Autodesk Fusion 360 part; units mm, degrees
(part 6 of 7)
  arc A999 (-78.9866, -79.4177) -> (-78.4866, -79.9177) centre (-78.4866, -79.4177) ccw
  line L1039 (33.4322, -41.8177) -> (46.4322, -41.8177)
  arc A1000 (208.3572, -60.8677) -> (208.8572, -60.3677) centre (208.3572, -60.3677) ccw
  line L1040 (-78.4866, -65.9177) -> (-65.4866, -65.9177)
  arc A1001 (-50.6991, -85.4677) -> (-51.1991, -84.9677) centre (-51.1991, -85.4677) ccw
  arc A1002 (27.3822, -41.8177) -> (27.8822, -41.3177) centre (27.3822, -41.3177) ccw
  arc A1003 (113.6072, -9.2677) -> (113.1072, -8.7677) centre (113.1072, -9.2677) ccw
  arc A1004 (-48.0303, -79.4177) -> (-47.5303, -79.9177) centre (-47.5303, -79.4177) ccw
  line L1041 (46.9322, -28.3177) -> (46.9322, -41.3177)
  arc A1005 (-20.2428, -3.7177) -> (-19.7428, -3.2177) centre (-20.2428, -3.2177) ccw
  line L1042 (4.0697, -66.4177) -> (4.0697, -79.4177)
  arc A1006 (75.7947, -60.3677) -> (76.2947, -60.8677) centre (76.2947, -60.3677) ccw
  arc A1007 (4.0697, -66.4177) -> (3.5697, -65.9177) centre (3.5697, -66.4177) ccw
  arc A1008 (194.8572, -98.4677) -> (195.3572, -98.9677) centre (195.3572, -98.4677) ccw
  line L1043 (80.5572, 9.7823) -> (80.5572, -3.2177)
  line L1044 (4.3572, 9.7823) -> (4.3572, -3.2177)
  line L1045 (27.8822, -28.3177) -> (27.8822, -41.3177)
  line L1046 (-63.0486, -66.9177) -> (-57.0486, -66.9177)
  arc A1009 (61.5072, -3.2177) -> (62.0072, -3.7177) centre (62.0072, -3.2177) ccw
  arc A1010 (-51.1991, -98.9677) -> (-50.6991, -98.4677) centre (-51.1991, -98.4677) ccw
  line L1047 (-8.9491, -86.4677) -> (-8.9491, -100.4677)
  line L1048 (175.8072, -66.4177) -> (175.8072, -79.4177)
  arc A1011 (84.5509, -85.9677) -> (84.0509, -86.4677) centre (84.5509, -86.4677) ccw
  arc A1012 (94.5572, -9.2677) -> (94.0572, -8.7677) centre (94.0572, -9.2677) ccw
  line L1049 (166.7822, -22.7677) -> (179.7822, -22.7677)
  line L1050 (176.3072, -98.9677) -> (189.3072, -98.9677)
  line L1051 (66.7697, -79.9177) -> (79.7697, -79.9177)
  line L1052 (195.3572, -60.8677) -> (208.3572, -60.8677)
  arc A1013 (-14.1928, 10.2823) -> (-14.6928, 9.7823) centre (-14.1928, 9.7823) ccw
  arc A1014 (100.1072, 10.2823) -> (99.6072, 9.7823) centre (100.1072, 9.7823) ccw
  arc A1015 (81.0572, 10.2823) -> (80.5572, 9.7823) centre (81.0572, 9.7823) ccw
  line L1053 (-0.6928, 9.7823) -> (-0.6928, -3.2177)
  line L1054 (137.7072, -9.2677) -> (137.7072, -22.2677)
  line L1055 (157.2572, -98.9677) -> (170.2572, -98.9677)
  line L1056 (179.8389, -62.8677) -> (185.8389, -62.8677)
  arc A1016 (62.0072, 10.2823) -> (61.5072, 9.7823) centre (62.0072, 9.7823) ccw
  arc A1017 (-78.4866, -65.9177) -> (-78.9866, -66.4177) centre (-78.4866, -66.4177) ccw
  line L1057 (33.4322, -27.8177) -> (46.4322, -27.8177)
  arc A1018 (-19.4553, -60.3677) -> (-18.9553, -60.8677) centre (-18.9553, -60.3677) ccw
  arc A1019 (9.6197, -65.9177) -> (9.1197, -66.4177) centre (9.6197, -66.4177) ccw
  line L1058 (84.5509, -100.9677) -> (90.5509, -100.9677)
  line L1059 (-83.2491, -60.8677) -> (-70.2491, -60.8677)
  arc A1020 (119.1572, 10.2823) -> (118.6572, 9.7823) centre (119.1572, 9.7823) ccw
  arc A1021 (-47.5303, -65.9177) -> (-48.0303, -66.4177) centre (-47.5303, -66.4177) ccw
  arc A1022 (23.4072, -22.2677) -> (23.9072, -22.7677) centre (23.9072, -22.2677) ccw
  arc A1023 (127.3947, -60.8677) -> (127.8947, -60.3677) centre (127.3947, -60.3677) ccw
  line L1060 (118.6572, -9.2677) -> (118.6572, -22.2677)
  line L1061 (62.0072, 10.2823) -> (75.0072, 10.2823)
  line L1062 (175.8072, -85.4677) -> (175.8072, -98.4677)
  line L1063 (-14.6928, 9.7823) -> (-14.6928, -3.2177)
  arc A1024 (113.8947, -60.3677) -> (114.3947, -60.8677) centre (114.3947, -60.3677) ccw
  arc A1025 (32.6447, -47.3677) -> (32.1447, -46.8677) centre (32.1447, -47.3677) ccw
  arc A1026 (185.8389, -62.8677) -> (186.3389, -62.3677) centre (185.8389, -62.3677) ccw
  line L1064 (90.0822, -28.3177) -> (90.0822, -41.3177)
  line L1065 (99.6072, -85.4677) -> (99.6072, -98.4677)
  line L1066 (195.3572, -98.9677) -> (208.3572, -98.9677)
  line L1067 (-52.2928, -8.7677) -> (-39.2928, -8.7677)
  arc A1027 (80.5572, -22.2677) -> (81.0572, -22.7677) centre (81.0572, -22.2677) ccw
  line L1068 (-14.1928, 10.2823) -> (-1.1928, 10.2823)
  arc A1028 (113.6072, 9.7823) -> (113.1072, 10.2823) centre (113.1072, 9.7823) ccw
  arc A1029 (38.1947, -46.8677) -> (37.6947, -47.3677) centre (38.1947, -47.3677) ccw
  arc A1030 (-40.3866, -84.9677) -> (-40.8866, -85.4677) centre (-40.3866, -85.4677) ccw
  line L1069 (85.3197, -66.4177) -> (85.3197, -79.4177)
  arc A1031 (132.1572, -98.9677) -> (132.6572, -98.4677) centre (132.1572, -98.4677) ccw
  arc A1032 (46.4322, -41.8177) -> (46.9322, -41.3177) centre (46.4322, -41.3177) ccw
  line L1070 (150.1134, -65.9177) -> (163.1134, -65.9177)
  line L1071 (176.3072, -79.9177) -> (189.3072, -79.9177)
  line L1072 (113.6072, -9.2677) -> (113.6072, -22.2677)
  arc A1033 (-57.5553, -60.3677) -> (-57.0553, -60.8677) centre (-57.0553, -60.3677) ccw
  arc A1034 (75.0072, -22.7677) -> (75.5072, -22.2677) centre (75.0072, -22.2677) ccw
  arc A1035 (52.4822, -27.8177) -> (51.9822, -28.3177) centre (52.4822, -28.3177) ccw
  arc A1036 (179.3389, -62.3677) -> (179.8389, -62.8677) centre (179.8389, -62.3677) ccw
  arc A1037 (113.1072, -3.7177) -> (113.6072, -3.2177) centre (113.1072, -3.2177) ccw
  arc A1038 (-38.5053, -60.3677) -> (-38.0053, -60.8677) centre (-38.0053, -60.3677) ccw
  arc A1039 (157.2572, -84.9677) -> (156.7572, -85.4677) centre (157.2572, -85.4677) ccw
  arc A1040 (94.5572, 9.7823) -> (94.0572, 10.2823) centre (94.0572, 9.7823) ccw
  arc A1041 (46.9322, -28.3177) -> (46.4322, -27.8177) centre (46.4322, -28.3177) ccw
  arc A1042 (-52.2928, 10.2823) -> (-52.7928, 9.7823) centre (-52.2928, 9.7823) ccw
  arc A1043 (-70.2491, -60.8677) -> (-69.7491, -60.3677) centre (-70.2491, -60.3677) ccw
  arc A1044 (-14.1928, -8.7677) -> (-14.6928, -9.2677) centre (-14.1928, -9.2677) ccw
  arc A1045 (189.8072, -85.4677) -> (189.3072, -84.9677) centre (189.3072, -85.4677) ccw
  arc A1046 (-34.5303, -79.9177) -> (-34.0303, -79.4177) centre (-34.5303, -79.4177) ccw
  arc A1047 (75.5072, -9.2677) -> (75.0072, -8.7677) centre (75.0072, -9.2677) ccw
  line L1073 (113.6072, 9.7823) -> (113.6072, -3.2177)
  arc A1048 (-0.6928, 9.7823) -> (-1.1928, 10.2823) centre (-1.1928, 9.7823) ccw
  arc A1049 (208.8572, -85.4677) -> (208.3572, -84.9677) centre (208.3572, -85.4677) ccw
  arc A1050 (136.9197, -79.9177) -> (137.4197, -79.4177) centre (136.9197, -79.4177) ccw
  arc A1051 (65.9822, -28.3177) -> (65.4822, -27.8177) centre (65.4822, -28.3177) ccw
  arc A1052 (75.0072, -3.7177) -> (75.5072, -3.2177) centre (75.0072, -3.2177) ccw
  arc A1053 (-15.9491, -100.4677) -> (-15.4491, -100.9677) centre (-15.4491, -100.4677) ccw
  line L1074 (114.3947, -60.8677) -> (127.3947, -60.8677)
  arc A1054 (195.3572, -84.9677) -> (194.8572, -85.4677) centre (195.3572, -85.4677) ccw
  arc A1055 (123.4197, -79.4177) -> (123.9197, -79.9177) centre (123.9197, -79.4177) ccw
  arc A1056 (-9.4303, -65.9177) -> (-9.9303, -66.4177) centre (-9.4303, -66.4177) ccw
  line L1075 (94.5572, -9.2677) -> (94.5572, -22.2677)
  line L1076 (4.3572, -9.2677) -> (4.3572, -22.2677)
  line L1077 (-74.5116, -85.4677) -> (-74.5116, -98.4677)
  arc A1057 (30.5509, -98.4677) -> (31.0509, -98.9677) centre (31.0509, -98.4677) ccw
  arc A1058 (42.4572, -22.2677) -> (42.9572, -22.7677) centre (42.9572, -22.2677) ccw
  arc A1059 (-15.4491, -85.9677) -> (-15.9491, -86.4677) centre (-15.4491, -86.4677) ccw
  line L1078 (-61.8178, -41.8177) -> (-48.8178, -41.8177)
  line L1079 (158.3442, -9.7677) -> (164.3442, -9.7677)
  line L1080 (-63.5486, -67.4177) -> (-63.5486, -81.4177)
  line L1081 (194.8572, -85.4677) -> (194.8572, -98.4677)
  line L1082 (42.1697, -66.4177) -> (42.1697, -79.4177)
  line L1083 (99.6072, 9.7823) -> (99.6072, -3.2177)
  arc A1060 (100.1072, -8.7677) -> (99.6072, -9.2677) centre (100.1072, -9.2677) ccw
  arc A1061 (-57.8428, -9.2677) -> (-58.3428, -8.7677) centre (-58.3428, -9.2677) ccw
  arc A1062 (-34.0303, -66.4177) -> (-34.5303, -65.9177) centre (-34.5303, -66.4177) ccw
  arc A1063 (-88.5116, -98.4677) -> (-88.0116, -98.9677) centre (-88.0116, -98.4677) ccw
  arc A1064 (123.9197, -65.9177) -> (123.4197, -66.4177) centre (123.9197, -66.4177) ccw
  line L1084 (75.5072, -9.2677) -> (75.5072, -22.2677)
  line L1085 (38.1947, -46.8677) -> (51.1947, -46.8677)
  arc A1065 (176.3072, -65.9177) -> (175.8072, -66.4177) centre (176.3072, -66.4177) ccw
  line L1086 (-88.0116, -84.9677) -> (-75.0116, -84.9677)
  line L1087 (-40.8866, -85.4677) -> (-40.8866, -98.4677)
  line L1088 (118.3697, -66.4177) -> (118.3697, -79.4177)
  arc A1066 (151.2072, -3.7177) -> (151.7072, -3.2177) centre (151.2072, -3.2177) ccw
  arc A1067 (22.6197, -79.9177) -> (23.1197, -79.4177) centre (22.6197, -79.4177) ccw
  arc A1068 (-80.4246, -67.4177) -> (-80.9246, -66.9177) centre (-80.9246, -67.4177) ccw
  line L1089 (18.3572, -9.2677) -> (18.3572, -22.2677)
  line L1090 (-26.8866, -85.4677) -> (-26.8866, -98.4677)
  arc A1069 (155.4629, -62.3677) -> (155.9629, -62.8677) centre (155.9629, -62.3677) ccw
  arc A1070 (119.1572, -8.7677) -> (118.6572, -9.2677) centre (119.1572, -9.2677) ccw
  arc A1071 (-39.2928, -3.7177) -> (-38.7928, -3.2177) centre (-39.2928, -3.2177) ccw
  line L1091 (31.0509, -98.9677) -> (44.0509, -98.9677)
  line L1092 (-64.9866, -66.4177) -> (-64.9866, -79.4177)
  line L1093 (-87.4246, -67.4177) -> (-87.4246, -81.4177)
  arc A1072 (17.8572, -22.7677) -> (18.3572, -22.2677) centre (17.8572, -22.2677) ccw
  arc A1073 (-83.7491, -60.3677) -> (-83.2491, -60.8677) centre (-83.2491, -60.3677) ccw
  arc A1074 (108.3447, -60.8677) -> (108.8447, -60.3677) centre (108.3447, -60.3677) ccw
  line L1094 (176.3072, -65.9177) -> (189.3072, -65.9177)
  line L1095 (151.7072, 9.7823) -> (151.7072, -3.2177)
  line L1096 (-15.9491, -86.4677) -> (-15.9491, -100.4677)
  arc A1075 (-52.2928, -8.7677) -> (-52.7928, -9.2677) centre (-52.2928, -9.2677) ccw
  line L1097 (-15.4491, -100.9677) -> (-9.4491, -100.9677)
  line L1098 (44.5509, -85.4677) -> (44.5509, -98.4677)
  arc A1076 (57.2447, -46.8677) -> (56.7447, -47.3677) centre (57.2447, -47.3677) ccw
  arc A1077 (85.3197, -79.4177) -> (85.8197, -79.9177) centre (85.8197, -79.4177) ccw
  line L1099 (-48.0303, -66.4177) -> (-48.0303, -79.4177)
  line L1100 (80.5572, -9.2677) -> (80.5572, -22.2677)
  arc A1078 (-15.4803, -79.9177) -> (-14.9803, -79.4177) centre (-15.4803, -79.4177) ccw
  line L1101 (56.4572, -9.2677) -> (56.4572, -22.2677)
  line L1102 (138.2072, 10.2823) -> (151.2072, 10.2823)
  arc A1079 (-74.5116, -85.4677) -> (-75.0116, -84.9677) centre (-75.0116, -85.4677) ccw
  line L1103 (156.7572, 9.7823) -> (156.7572, -3.2177)
  line L1104 (47.2197, -66.4177) -> (47.2197, -79.4177)
  arc A1080 (9.1197, -79.4177) -> (9.6197, -79.9177) centre (9.6197, -79.4177) ccw
  arc A1081 (44.0509, -98.9677) -> (44.5509, -98.4677) centre (44.0509, -98.4677) ccw
  line L1105 (-50.6991, -85.4677) -> (-50.6991, -98.4677)
  arc A1082 (118.6572, -3.2177) -> (119.1572, -3.7177) centre (119.1572, -3.2177) ccw
  line L1106 (100.1072, -8.7677) -> (113.1072, -8.7677)
  line L1107 (104.3697, -66.4177) -> (104.3697, -79.4177)
  arc A1083 (4.8572, -8.7677) -> (4.3572, -9.2677) centre (4.8572, -9.2677) ccw
  line L1108 (186.3389, -48.3677) -> (186.3389, -62.3677)
  arc A1084 (99.6072, -3.2177) -> (100.1072, -3.7177) centre (100.1072, -3.2177) ccw
  arc A1085 (118.3697, -66.4177) -> (117.8697, -65.9177) centre (117.8697, -66.4177) ccw
  line L1109 (28.6697, -65.9177) -> (41.6697, -65.9177)
  arc A1086 (60.7197, -79.9177) -> (61.2197, -79.4177) centre (60.7197, -79.4177) ccw
  arc A1087 (151.7072, 9.7823) -> (151.2072, 10.2823) centre (151.2072, 9.7823) ccw
  arc A1088 (51.1947, -60.8677) -> (51.6947, -60.3677) centre (51.1947, -60.3677) ccw
  arc A1089 (117.8697, -79.9177) -> (118.3697, -79.4177) centre (117.8697, -79.4177) ccw
  arc A1090 (-40.8866, -98.4677) -> (-40.3866, -98.9677) centre (-40.3866, -98.4677) ccw
  arc A1091 (-33.2428, 10.2823) -> (-33.7428, 9.7823) centre (-33.2428, 9.7823) ccw
  arc A1092 (66.2697, -79.4177) -> (66.7697, -79.9177) centre (66.7697, -79.4177) ccw
  line L1110 (157.2572, 10.2823) -> (170.2572, 10.2823)
  arc A1093 (176.3072, -84.9677) -> (175.8072, -85.4677) centre (176.3072, -85.4677) ccw
  arc A1094 (-64.1991, -84.9677) -> (-64.6991, -85.4677) centre (-64.1991, -85.4677) ccw
  arc A1095 (-64.9866, -66.4177) -> (-65.4866, -65.9177) centre (-65.4866, -66.4177) ccw
  line L1111 (-80.4246, -67.4177) -> (-80.4246, -81.4177)
  arc A1096 (3.5697, -79.9177) -> (4.0697, -79.4177) centre (3.5697, -79.4177) ccw
  arc A1097 (-58.3428, -3.7177) -> (-57.8428, -3.2177) centre (-58.3428, -3.2177) ccw
  arc A1098 (-28.4803, -65.9177) -> (-28.9803, -66.4177) centre (-28.4803, -66.4177) ccw
  line L1112 (100.1072, -3.7177) -> (113.1072, -3.7177)
  arc A1099 (-5.9553, -60.8677) -> (-5.4553, -60.3677) centre (-5.9553, -60.3677) ccw
  arc A1100 (-88.0116, -84.9677) -> (-88.5116, -85.4677) centre (-88.0116, -85.4677) ccw
  line L1113 (37.4072, -9.2677) -> (37.4072, -22.2677)
  arc A1101 (51.6947, -47.3677) -> (51.1947, -46.8677) centre (51.1947, -47.3677) ccw
  arc A1102 (19.1447, -46.8677) -> (18.6447, -47.3677) centre (19.1447, -47.3677) ccw
  arc A1103 (51.9822, -41.3177) -> (52.4822, -41.8177) centre (52.4822, -41.3177) ccw
  line L1114 (99.3197, -66.4177) -> (99.3197, -79.4177)
  line L1115 (-19.7428, -9.2677) -> (-19.7428, -22.2677)
  line L1116 (-103.7226, 22.4007) -> (218.9474, 22.4007)
  line L1117 (218.9474, 22.4007) -> (218.9474, -108.8427)
  line L1118 (218.9474, -108.8427) -> (-103.7226, -108.8427)
  line L1119 (-103.7226, -108.8427) -> (-103.7226, 22.4007)
  circle A1104 centre (-107.7226, 51.4273) radius 1.75
  circle A1105 centre (-107.7226, -112.8427) radius 1.75
  circle A1106 centre (222.9474, 51.4273) radius 1.75
  circle A1107 centre (222.9474, -112.8427) radius 1.75
  dimension "d1" = 25.211
  dimension "d2" = 19.875
  dimension "d3" = 25.211
  dimension "d4" = 19.875
  dimension "d5" = 25.211
  dimension "d6" = 19.875
  dimension "d8" = 10
  dimension "d9" = 10
  dimension "d10" = 10
  dimension "d11" = 3.5
  dimension "d12" = 6
  dimension "d13" = 6
  dimension "d14" = 3.5
  dimension "d15" = 6
  dimension "d16" = 6
  dimension "d17" = 3.5
  dimension "d18" = 6
  dimension "d19" = 6
  dimension "d20" = 3.5
  dimension "d21" = 6
  dimension "d22" = 6
  constraint horizontal L40
  constraint vertical L60
  constraint horizontal L155
  constraint vertical L18
  constraint horizontal L412
  constraint vertical L432
  constraint horizontal L527
  constraint vertical L390
  constraint horizontal L784
  constraint vertical L804
  constraint horizontal L899
  constraint vertical L762
  constraint horizontal L1116
  constraint vertical L1117
  constraint horizontal L1118
  constraint vertical L1119
  measures "d1" distance of L18 L112
  measures "d2" distance of L100 L155
  measures "d3" distance of L390 L484
  measures "d4" distance of L472 L527
  measures "d5" distance of L762 L856
  measures "d6" distance of L844 L899
  measures "d8" distance of L762 L1119
  measures "d9" distance of L804 L1117
  measures "d10" distance of L527 L1118
  measures "d11" diameter of A1107
  measures "d12" distance of L804 A1107.centre
  measures "d13" distance of L899 A1107.centre
  measures "d14" diameter of A1106
  measures "d15" distance of L60 A1106.centre
  measures "d16" distance of L784 A1106.centre
  measures "d17" diameter of A1104
  measures "d18" distance of L412 A1104.centre
  measures "d19" distance of L762 A1104.centre
  measures "d20" diameter of A1105
  measures "d21" distance of L527 A1105.centre
  measures "d22" distance of L18 A1105.centre
extrude "Extrude1" add sketch "Sketch1" along normal blind 6 contours L18 L40 L60 L155 L390 L412 L432 L527 L762 L784 L804 L899 makes body 1
fillet "Fillet1" radius 9 4 edges at (-113.7226, -118.8427, 3) (-113.7226, 57.4273, 3) (228.9474, 57.4273, 3) (228.9474, -118.8427, 3) on bodies 1
fillet "Fillet2" radius 5 4 edges at (218.9474, 22.4007, 3) (-103.7226, 22.4007, 3) (-103.7226, -108.8427, 3) (218.9474, -108.8427, 3) on bodies 1
sketch "Sketch2" plane through (0, 0, 6) normal (0, 0, 1) x (-1, 0, 0)
  arc A0 (-219.9474, 118.8427) -> (-228.9474, 109.8427) centre (-219.9474, 109.8427) ccw
  line L0 (-228.9474, 109.8427) -> (-228.9474, -48.4273)
  arc A1 (-228.9474, -48.4273) -> (-219.9474, -57.4273) centre (-219.9474, -48.4273) ccw
  line L1 (-219.9474, -57.4273) -> (104.7226, -57.4273)
  arc A2 (104.7226, -57.4273) -> (113.7226, -48.4273) centre (104.7226, -48.4273) ccw
  line L2 (113.7226, -48.4273) -> (113.7226, 109.8427)
  arc A3 (113.7226, 109.8427) -> (104.7226, 118.8427) centre (104.7226, 109.8427) ccw
  line L3 (104.7226, 118.8427) -> (-219.9474, 118.8427)
  circle A4 centre (107.7226, 112.8427) radius 1.75
  circle A5 centre (-222.9474, 112.8427) radius 1.75
  circle A6 centre (-222.9474, -51.4273) radius 1.75
  line L4 (-213.9474, 108.8427) -> (98.7226, 108.8427)
  arc A7 (103.7226, 103.8427) -> (98.7226, 108.8427) centre (98.7226, 103.8427) ccw
  line L5 (103.7226, 103.8427) -> (103.7226, -17.4007)
  arc A8 (98.7226, -22.4007) -> (103.7226, -17.4007) centre (98.7226, -17.4007) ccw
  line L6 (98.7226, -22.4007) -> (-213.9474, -22.4007)
  arc A9 (-218.9474, -17.4007) -> (-213.9474, -22.4007) centre (-213.9474, -17.4007) ccw
  line L7 (-218.9474, -17.4007) -> (-218.9474, 103.8427)
  arc A10 (-213.9474, 108.8427) -> (-218.9474, 103.8427) centre (-213.9474, 103.8427) ccw
  circle A11 centre (107.7226, -51.4273) radius 1.75
  line L8 (110, -40) -> (110, 105)
  line L9 (108, 105) -> (108, 96)
  line L10 (108, 96) -> (106.5, 95)
  line L11 (106.5, 95) -> (106.5, 90)
  line L12 (106.5, 90) -> (108, 88.6859)
  line L13 (108, 88.6859) -> (108, 59)
  line L14 (108, 59) -> (106, 58)
  line L15 (106, 58) -> (106, 28)
  line L16 (106, 28) -> (108, 24)
  line L17 (108, 24) -> (108, -19)
  line L18 (108, -19) -> (107, -21)
  line L19 (107, -21) -> (105, -21)
  line L20 (105, -21) -> (104, -23)
  line L21 (104, -23) -> (102, -23)
  line L22 (102, -23) -> (101, -25)
  line L23 (101, -25) -> (97, -25)
  line L24 (97, -25) -> (95, -27)
  line L25 (95, -27) -> (95, -30)
  line L26 (95, -30) -> (95, -37.2329)
  line L27 (95, -37.2329) -> (94.9816, -37.2145)
  line L28 (110, -40) -> (110, -45)
  line L29 (110, -45) -> (107, -46)
  line L30 (107, -46) -> (104.7226, -46.7591)
  line L31 (104.7226, -46.7591) -> (99.718, -48.4273)
  line L32 (99.718, -48.4273) -> (99.718, -51)
  line L33 (99.718, -51) -> (55, -51)
  line L34 (55, -51) -> (53.023, -52.318)
  line L35 (53.023, -52.318) -> (24.5454, -52.318)
  line L36 (24.5454, -52.318) -> (23.6667, -51)
  line L37 (23.6667, -51) -> (-31, -51)
  line L38 (-31, -51) -> (-80, -51)
  line L39 (-80, -51) -> (-83, -54)
  line L40 (-83, -54) -> (-120, -54)
  line L41 (-120, -54) -> (-122, -51)
  line L42 (-122, -51) -> (-200, -51)
  line L43 (-200, -51) -> (-204.3677, -48.4273)
  line L44 (-204.3677, -48.4273) -> (-209, -48.4273)
  line L45 (-209, -48.4273) -> (-212.364, -46.4459)
  line L46 (-212.364, -46.4459) -> (-216, -46.4459)
  line L47 (-216, -46.4459) -> (-218.7538, -44.8239)
  line L48 (-218.7538, -44.8239) -> (-223, -44.8239)
  line L49 (-223, -44.8239) -> (-224.9863, -43.6539)
  line L50 (-224.9863, -43.6539) -> (-224.9863, -21)
  line L51 (-224.9863, -21) -> (-227, -19)
  line L52 (-227, -19) -> (-227, -10)
  line L53 (-227, -10) -> (-224.9863, -6.5812)
  line L54 (-224.9863, -6.5812) -> (-224.9863, 40)
  line L55 (-224.9863, 40) -> (-227, 43.4506)
  line L56 (-227, 43.4506) -> (-227, 75)
  line L57 (-227, 75) -> (-224.9863, 77.9634)
  line L58 (-224.9863, 77.9634) -> (-224.9863, 105)
  line L59 (-224.9863, 105) -> (-224.9863, 107.3782)
  line L60 (-224.9863, 107.3782) -> (-222, 108)
  line L61 (-222, 108) -> (-219.9474, 109.8427)
  line L62 (-219.9474, 109.8427) -> (-217.5, 112.5)
  line L63 (-217.5, 112.5) -> (-215, 115)
  line L64 (-215, 115) -> (-111.4311, 115)
  line L65 (-111.4311, 115) -> (-99, 115)
  line L66 (-99, 115) -> (-97.0321, 116.7667)
  line L67 (-97.0321, 116.7667) -> (-32.7128, 116.7667)
  line L68 (-32.7128, 116.7667) -> (-30, 115)
  line L69 (-30, 115) -> (100, 115)
  line L70 (100, 115) -> (102.1243, 112.8427)
  line L71 (102.1243, 112.8427) -> (104.0883, 112.4123)
  line L72 (104.0883, 112.4123) -> (105.5565, 110.9212)
  line L73 (105.5565, 110.9212) -> (107.1244, 109.329)
  line L74 (107.1244, 109.329) -> (110, 109.329)
  line L75 (110, 109.329) -> (110, 105)
  line L76 (108, 105) -> (108, 107)
  line L77 (108, 107) -> (105, 107)
  line L78 (105, 107) -> (103, 110)
  line L79 (103, 110) -> (101, 111)
  line L80 (101, 111) -> (98.9961, 113.0039)
  line L81 (98.9961, 113.0039) -> (78.0039, 113.0039)
  line L82 (78.0039, 113.0039) -> (76, 111)
  line L83 (76, 111) -> (58, 111)
  line L84 (58, 111) -> (56, 113)
  line L85 (56, 113) -> (12, 113)
  line L86 (12, 113) -> (10, 111)
  line L87 (10, 111) -> (0, 111)
  line L88 (0, 111) -> (-2, 113)
  line L89 (-2, 113) -> (-105, 113)
  line L90 (-105, 113) -> (-140, 113)
  line L91 (-140, 113) -> (-195, 113)
  line L92 (-195, 113) -> (-197, 111)
  line L93 (-197, 111) -> (-206, 111)
  line L94 (-206, 111) -> (-207.5, 112.5)
  line L95 (-207.5, 112.5) -> (-208, 113)
  line L96 (-208, 113) -> (-214, 113)
  line L97 (-214, 113) -> (-215, 113)
  line L98 (-215, 113) -> (-218.9474, 109.0526)
  line L99 (-218.9474, 109.0526) -> (-221.3805, 106.6195)
  line L100 (-221.3805, 106.6195) -> (-223, 106)
  line L101 (-223, 106) -> (-223, 35)
  line L102 (-223, 35) -> (-222, 34)
  line L103 (-222, 34) -> (-222, 8.6485)
  line L104 (-222, 8.6485) -> (-223, 7)
  line L105 (-223, 7) -> (-223, -36.5124)
  line L106 (-223, -36.5124) -> (-218.7538, -40.3244)
  line L107 (-218.7538, -40.3244) -> (-214.9132, -42.5866)
  line L108 (-214.9132, -42.5866) -> (-209, -42.5866)
  line L109 (-209, -42.5866) -> (-206.5079, -44.8239)
  line L110 (-206.5079, -44.8239) -> (-203, -44.8239)
  line L111 (-203, -44.8239) -> (-198, -49)
  line L112 (-198, -49) -> (-166, -49)
  line L113 (-166, -49) -> (-164.1255, -46.9119)
  line L114 (-164.1255, -46.9119) -> (-144, -46.9119)
  line L115 (-144, -46.9119) -> (-141.6741, -49)
  line L116 (-141.6741, -49) -> (-55, -49)
  line L117 (-55, -49) -> (-53.1255, -46.9119)
  line L118 (-53.1255, -46.9119) -> (-7, -46.9119)
  line L119 (-7, -46.9119) -> (-5, -49)
  line L120 (-5, -49) -> (90.0217, -49)
  line L121 (90.0217, -49) -> (95.0077, -45.5)
  line L122 (95.0077, -45.5) -> (95.0077, -45.4411)
  line L123 (95.0077, -45.4411) -> (94.9816, -37.2145)
  line L124 (79.9728, -47.0166) -> (85.4987, -44.6483)
  line L125 (85.4987, -44.6483) -> (85.4987, -43.6179)
  line L126 (85.4987, -43.6179) -> (79.9839, -45.9814)
  line L127 (79.9728, -47.0166) -> (79.9839, -45.9814) construction
  line L128 (79.9728, -47.0166) -> (74.4988, -44.5304)
  line L129 (74.4988, -44.5304) -> (74.5209, -43.5002)
  line L130 (74.5209, -43.5002) -> (79.9839, -45.9814)
  line L131 (80.0522, -44.5759) -> (74.5262, -42.2076)
  line L132 (80.0522, -44.5759) -> (85.5261, -42.0897)
  line L133 (85.504, -41.0595) -> (80.0411, -43.5407)
  line L134 (85.5261, -42.0897) -> (85.504, -41.0595)
  line L135 (74.5262, -41.1772) -> (80.0411, -43.5407)
  line L136 (74.5262, -42.2076) -> (74.5262, -41.1772)
  line L137 (79.9047, -39.8001) -> (74.4308, -37.3139)
  line L138 (85.4307, -37.4319) -> (85.4307, -36.4015)
  line L139 (79.9047, -39.8001) -> (85.4307, -37.4319)
  line L140 (85.4581, -39.7547) -> (85.436, -38.7245)
  line L141 (74.4308, -37.3139) -> (74.4529, -36.2838)
  line L142 (85.436, -38.7245) -> (79.9731, -41.2057)
  line L143 (74.4529, -36.2838) -> (79.9158, -38.765)
  line L144 (79.9842, -42.2409) -> (85.4581, -39.7547)
  line L145 (74.4582, -39.8726) -> (74.4582, -38.8422)
  line L146 (85.4307, -36.4015) -> (79.9158, -38.765)
  line L147 (79.9842, -42.2409) -> (74.4582, -39.8726)
  line L148 (79.9842, -42.2409) -> (79.9731, -41.2057) construction
  line L149 (74.4582, -38.8422) -> (79.9731, -41.2057)
  line L150 (85.4987, -47.4996) -> (85.4987, -25.2234) construction
  line L151 (79.8932, -32.8108) -> (79.9043, -31.7757) construction
  line L152 (74.3733, -31.6295) -> (79.8362, -34.1107)
  line L153 (74.3786, -35.2183) -> (74.3786, -34.1879)
  line L154 (79.8251, -35.1458) -> (85.3511, -32.7776)
  line L155 (74.3786, -34.1879) -> (79.8935, -36.5514)
  line L156 (79.8932, -32.8108) -> (74.4193, -30.3246)
  line L157 (74.3512, -32.6596) -> (74.3733, -31.6295)
  line L158 (79.9046, -37.5866) -> (85.3785, -35.1004)
  line L159 (79.8932, -32.8108) -> (85.4192, -30.4426)
  line L160 (85.3511, -31.7472) -> (79.8362, -34.1107)
  line L161 (85.3511, -32.7776) -> (85.3511, -31.7472)
  line L162 (79.9046, -37.5866) -> (79.8935, -36.5514) construction
  line L163 (85.4192, -30.4426) -> (85.4192, -29.4122)
  line L164 (74.4414, -29.2945) -> (79.9043, -31.7757)
  line L165 (85.3785, -35.1004) -> (85.3564, -34.0702)
  line L166 (74.4467, -26.9714) -> (79.9615, -29.335)
  line L167 (79.9726, -30.3701) -> (74.4467, -28.0018)
  line L168 (79.8251, -35.1458) -> (74.3512, -32.6596)
  line L169 (85.4466, -27.8839) -> (85.4245, -26.8538)
  line L170 (85.3564, -34.0702) -> (79.8935, -36.5514)
  line L171 (79.9046, -37.5866) -> (74.3786, -35.2183)
  line L172 (79.9726, -30.3701) -> (85.4466, -27.8839)
  line L173 (85.4245, -26.8538) -> (79.9615, -29.335)
  line L174 (74.4193, -30.3246) -> (74.4414, -29.2945)
  line L175 (85.4192, -29.4122) -> (79.9043, -31.7757)
  line L176 (74.4467, -28.0018) -> (74.4467, -26.9714)
  line L177 (55, -46) -> (65, -30)
  line L178 (65, -30) -> (44, -30)
  line L179 (44, -30) -> (55, -46)
  line L180 (55, -48) -> (67, -29)
  line L181 (67, -29) -> (42, -29)
  line L182 (42, -29) -> (55, -48)
  line L183 (55.638, -43.2362) -> (54.2071, -43.2362)
  line L184 (54.2071, -43.2362) -> (54.2071, -33.9141)
  line L185 (54.2071, -33.9141) -> (55.638, -33.9141)
  line L186 (55.638, -33.9141) -> (55.638, -43.2362)
  circle A12 centre (54.9514, -32.4983) radius 0.8407
  line L187 (-144.2264, -40.7236) -> (-140.2264, -36.7236)
  line L188 (-140.2264, -36.7236) -> (-179.2264, -36.7236)
  line L189 (-179.2264, -36.7236) -> (-180.0146, -38.3)
  line L190 (-180.0146, -38.3) -> (-152.9, -38.3)
  line L191 (-152.9, -38.3) -> (-151.2264, -40.7236)
  line L192 (-151.2264, -40.7236) -> (-144.2264, -40.7236)
  line L193 (-153.2344, -39.0462) -> (-189.9389, -39.1613)
  line L194 (-189.9389, -39.1613) -> (-188.2093, -42.0152)
  line L195 (-188.2093, -42.0152) -> (-151.3887, -42.0152)
  line L196 (-151.3887, -42.0152) -> (-153.2344, -39.0462)
  line L197 (-137.6491, -35) -> (-178.2775, -35)
  line L198 (-178.2775, -35) -> (-182.1257, -37.5655)
  line L199 (-182.1257, -37.5655) -> (-200, -37.5655)
  line L200 (-200, -37.5655) -> (-200, -36.377)
  line L201 (-200, -36.377) -> (-182.5655, -36.377)
  line L202 (-182.5655, -36.377) -> (-179, -34)
  line L203 (-179, -34) -> (-138.1989, -34)
  line L204 (-138.1989, -34) -> (-135.1886, -29.1904)
  line L205 (-137.6491, -35) -> (-134.2833, -29.7167)
  line L206 (-134.2833, -29.7167) -> (-135.1886, -29.1904)
  line L207 (-143.8469, -32.9977) -> (-144.4496, -32.6498)
  line L208 (-144.4496, -32.6498) -> (-142.2994, -28.9256)
  line L209 (-142.2994, -28.9256) -> (-141.6968, -29.2736)
  line L210 (-141.6968, -29.2736) -> (-143.8469, -32.9977)
  line L211 (-142.2994, -28.9256) -> (-141.6968, -29.2736)
  line L212 (-144.4496, -32.6498) -> (-142.2994, -28.9256)
  line L213 (-141.6968, -29.2736) -> (-143.8469, -32.9977)
  line L214 (-143.8469, -32.9977) -> (-144.4496, -32.6498)
  line L215 (-143.3648, -29.2464) -> (-145.5149, -32.9705)
  line L216 (-143.9674, -28.8984) -> (-143.3648, -29.2464)
  line L217 (-143.9674, -28.8984) -> (-143.3648, -29.2464)
  line L218 (-143.3648, -29.2464) -> (-145.5149, -32.9705)
  line L219 (-145.5149, -32.9705) -> (-146.1175, -32.6226)
  line L220 (-146.1175, -32.6226) -> (-143.9674, -28.8984)
  line L221 (-146.5557, -29.2101) -> (-148.7058, -32.9343)
  line L222 (-144.8877, -29.2373) -> (-147.0378, -32.9615)
  line L223 (-145.4904, -28.8894) -> (-144.8877, -29.2373)
  line L224 (-147.6405, -32.6135) -> (-145.4904, -28.8894)
  line L225 (-145.4904, -28.8894) -> (-144.8877, -29.2373)
  line L226 (-147.0378, -32.9615) -> (-147.6405, -32.6135)
  line L227 (-147.0378, -32.9615) -> (-147.6405, -32.6135)
  line L228 (-144.8877, -29.2373) -> (-147.0378, -32.9615)
  line L229 (-147.1583, -28.8622) -> (-146.5557, -29.2101)
  line L230 (-147.1583, -28.8622) -> (-146.5557, -29.2101)
  line L231 (-147.6405, -32.6135) -> (-145.4904, -28.8894)
  line L232 (-146.5557, -29.2101) -> (-148.7058, -32.9343)
  line L233 (-148.7058, -32.9343) -> (-149.3085, -32.5863)
  line L234 (-149.3085, -32.5863) -> (-147.1583, -28.8622)
  line L235 (-152.7417, -32.59) -> (-150.5916, -28.8659)
  line L236 (-150.4711, -32.9652) -> (-151.0737, -32.6172)
  line L237 (-153.7825, -28.8297) -> (-153.1799, -29.1776)
  line L238 (-151.0737, -32.6172) -> (-148.9236, -28.8931)
  line L239 (-149.9889, -29.2139) -> (-152.1391, -32.938)
  line L240 (-150.5916, -28.8659) -> (-149.9889, -29.2139)
  line L241 (-150.5916, -28.8659) -> (-149.9889, -29.2139)
  line L242 (-152.1391, -32.938) -> (-152.7417, -32.59)
  line L243 (-155.33, -32.9017) -> (-155.9326, -32.5538)
  line L244 (-153.662, -32.9289) -> (-154.2647, -32.581)
  line L245 (-153.662, -32.9289) -> (-154.2647, -32.581)
  line L246 (-155.9326, -32.5538) -> (-153.7825, -28.8297)
  line L247 (-150.4711, -32.9652) -> (-151.0737, -32.6172)
  line L248 (-149.9889, -29.2139) -> (-152.1391, -32.938)
  line L249 (-151.0737, -32.6172) -> (-148.9236, -28.8931)
  line L250 (-153.7825, -28.8297) -> (-153.1799, -29.1776)
  line L251 (-153.1799, -29.1776) -> (-155.33, -32.9017)
  line L252 (-152.1145, -28.8569) -> (-151.5119, -29.2048)
  line L253 (-154.2647, -32.581) -> (-152.1145, -28.8569)
  line L254 (-154.2647, -32.581) -> (-152.1145, -28.8569)
  line L255 (-152.1145, -28.8569) -> (-151.5119, -29.2048)
  line L256 (-151.5119, -29.2048) -> (-153.662, -32.9289)
  line L257 (-153.1799, -29.1776) -> (-155.33, -32.9017)
  line L258 (-151.5119, -29.2048) -> (-153.662, -32.9289)
  line L259 (-148.321, -29.2411) -> (-150.4711, -32.9652)
  line L260 (-148.9236, -28.8931) -> (-148.321, -29.2411)
  line L261 (-160.2369, -28.8156) -> (-159.6342, -29.1636)
  line L262 (-165.1931, -28.8103) -> (-164.5904, -29.1582)
  line L263 (-166.7405, -32.8824) -> (-167.3432, -32.5344)
  line L264 (-166.8611, -28.7831) -> (-166.2584, -29.131)
  line L265 (-166.8611, -28.7831) -> (-166.2584, -29.131)
  line L266 (-161.7843, -32.8877) -> (-162.387, -32.5397)
  line L267 (-159.6342, -29.1636) -> (-161.7843, -32.8877)
  line L268 (-166.2584, -29.131) -> (-168.4085, -32.8552)
  line L269 (-156.9254, -32.9511) -> (-157.5281, -32.6032)
  line L270 (-158.5689, -28.8428) -> (-157.9662, -29.1908)
  line L271 (-157.9662, -29.1908) -> (-160.1164, -32.9149)
  line L272 (-159.6342, -29.1636) -> (-161.7843, -32.8877)
  line L273 (-160.1164, -32.9149) -> (-160.719, -32.5669)
  line L274 (-157.9662, -29.1908) -> (-160.1164, -32.9149)
  line L275 (-163.6701, -28.8193) -> (-163.0675, -29.1673)
  line L276 (-156.4433, -29.1998) -> (-158.5934, -32.9239)
  line L277 (-163.5496, -32.9186) -> (-164.1523, -32.5707)
  line L278 (-166.7405, -32.8824) -> (-167.3432, -32.5344)
  line L279 (-167.3432, -32.5344) -> (-165.1931, -28.8103)
  line L280 (-156.9254, -32.9511) -> (-157.5281, -32.6032)
  line L281 (-166.2584, -29.131) -> (-168.4085, -32.8552)
  line L282 (-167.3432, -32.5344) -> (-165.1931, -28.8103)
  line L283 (-157.5281, -32.6032) -> (-155.378, -28.8791)
  line L284 (-164.1523, -32.5707) -> (-162.0021, -28.8465)
  line L285 (-161.3995, -29.1945) -> (-163.5496, -32.9186)
  line L286 (-165.1931, -28.8103) -> (-164.5904, -29.1582)
  line L287 (-169.0112, -32.5072) -> (-166.8611, -28.7831)
  line L288 (-165.2176, -32.8914) -> (-165.8203, -32.5435)
  line L289 (-163.5496, -32.9186) -> (-164.1523, -32.5707)
  line L290 (-164.5904, -29.1582) -> (-166.7405, -32.8824)
  line L291 (-165.8203, -32.5435) -> (-163.6701, -28.8193)
  line L292 (-163.0675, -29.1673) -> (-165.2176, -32.8914)
  line L293 (-160.719, -32.5669) -> (-158.5689, -28.8428)
  line L294 (-160.719, -32.5669) -> (-158.5689, -28.8428)
  line L295 (-160.2369, -28.8156) -> (-159.6342, -29.1636)
  line L296 (-168.4085, -32.8552) -> (-169.0112, -32.5072)
  line L297 (-157.046, -28.8519) -> (-156.4433, -29.1998)
  line L298 (-157.5281, -32.6032) -> (-155.378, -28.8791)
  line L299 (-160.1164, -32.9149) -> (-160.719, -32.5669)
  line L300 (-164.1523, -32.5707) -> (-162.0021, -28.8465)
  line L301 (-158.5934, -32.9239) -> (-159.1961, -32.576)
  line L302 (-164.5904, -29.1582) -> (-166.7405, -32.8824)
  line L303 (-157.046, -28.8519) -> (-156.4433, -29.1998)
  line L304 (-156.4433, -29.1998) -> (-158.5934, -32.9239)
  line L305 (-159.1961, -32.576) -> (-157.046, -28.8519)
  line L306 (-162.387, -32.5397) -> (-160.2369, -28.8156)
  line L307 (-163.0675, -29.1673) -> (-165.2176, -32.8914)
  line L308 (-163.6701, -28.8193) -> (-163.0675, -29.1673)
  line L309 (-158.5689, -28.8428) -> (-157.9662, -29.1908)
  line L310 (-162.0021, -28.8465) -> (-161.3995, -29.1945)
  line L311 (-154.7753, -29.227) -> (-156.9254, -32.9511)
  line L312 (-155.378, -28.8791) -> (-154.7753, -29.227)
  line L313 (-180.4144, -32.4692) -> (-178.2643, -28.7451)
  line L314 (-178.2643, -28.7451) -> (-177.6617, -29.0931)
  line L315 (-182.0824, -32.4421) -> (-179.9323, -28.7179)
  line L316 (-171.6401, -28.7777) -> (-171.0375, -29.1256)
  line L317 (-190.7402, -29.0465) -> (-192.8903, -32.7706)
  line L318 (-193.493, -32.4227) -> (-191.3428, -28.6985)
  line L319 (-172.2673, -32.5108) -> (-170.1172, -28.7867)
  line L320 (-169.5145, -29.1347) -> (-171.6647, -32.8588)
  line L321 (-169.5145, -29.1347) -> (-171.6647, -32.8588)
  line L322 (-177.2235, -32.5055) -> (-175.0734, -28.7814)
  line L323 (-176.1387, -29.1021) -> (-178.2888, -32.8263)
  line L324 (-188.5368, -32.428) -> (-186.3866, -28.7039)
  line L325 (-175.4582, -32.4746) -> (-173.3081, -28.7505)
  line L326 (-174.4707, -29.1293) -> (-176.6209, -32.8535)
  line L327 (-186.8688, -32.4552) -> (-184.7187, -28.7311)
  line L328 (-178.2643, -28.7451) -> (-177.6617, -29.0931)
  line L329 (-169.9967, -32.886) -> (-170.5993, -32.538)
  line L330 (-174.8556, -32.8225) -> (-175.4582, -32.4746)
  line L331 (-176.6209, -32.8535) -> (-177.2235, -32.5055)
  line L332 (-188.1519, -28.7348) -> (-187.5493, -29.0828)
  line L333 (-176.7414, -28.7542) -> (-176.1387, -29.1021)
  line L334 (-175.0734, -28.7814) -> (-174.4707, -29.1293)
  line L335 (-170.1172, -28.7867) -> (-169.5145, -29.1347)
  line L336 (-179.9323, -28.7179) -> (-179.3296, -29.0659)
  line L337 (-170.1172, -28.7867) -> (-169.5145, -29.1347)
  line L338 (-181.4798, -32.79) -> (-182.0824, -32.4421)
  line L339 (-186.8688, -32.4552) -> (-184.7187, -28.7311)
  line L340 (-170.5993, -32.538) -> (-168.4492, -28.8139)
  line L341 (-173.1876, -32.8497) -> (-173.7903, -32.5018)
  line L342 (-193.493, -32.4227) -> (-191.3428, -28.6985)
  line L343 (-176.7414, -28.7542) -> (-176.1387, -29.1021)
  line L344 (-187.5493, -29.0828) -> (-189.6994, -32.8069)
  line L345 (-177.6617, -29.0931) -> (-179.8118, -32.8172)
  line L346 (-171.6647, -32.8588) -> (-172.2673, -32.5108)
  line L347 (-189.2172, -29.0556) -> (-191.3674, -32.7797)
  line L348 (-177.2235, -32.5055) -> (-175.0734, -28.7814)
  line L349 (-171.0375, -29.1256) -> (-173.1876, -32.8497)
  line L350 (-172.7055, -29.0984) -> (-174.8556, -32.8225)
  line L351 (-173.3081, -28.7505) -> (-172.7055, -29.0984)
  line L352 (-185.784, -29.0518) -> (-187.9341, -32.776)
  line L353 (-172.7055, -29.0984) -> (-174.8556, -32.8225)
  line L354 (-173.7903, -32.5018) -> (-171.6401, -28.7777)
  line L355 (-173.3081, -28.7505) -> (-172.7055, -29.0984)
  line L356 (-171.0375, -29.1256) -> (-173.1876, -32.8497)
  line L357 (-173.7903, -32.5018) -> (-171.6401, -28.7777)
  line L358 (-176.1387, -29.1021) -> (-178.2888, -32.8263)
  line L359 (-186.2661, -32.8032) -> (-186.8688, -32.4552)
  line L360 (-173.1876, -32.8497) -> (-173.7903, -32.5018)
  line L361 (-185.784, -29.0518) -> (-187.9341, -32.776)
  line L362 (-186.2661, -32.8032) -> (-186.8688, -32.4552)
  line L363 (-176.6209, -32.8535) -> (-177.2235, -32.5055)
  line L364 (-183.0752, -32.8394) -> (-183.6779, -32.4915)
  line L365 (-189.8199, -28.7076) -> (-189.2172, -29.0556)
  line L366 (-184.7187, -28.7311) -> (-184.116, -29.079)
  line L367 (-182.5931, -29.0881) -> (-184.7432, -32.8122)
  line L368 (-184.7187, -28.7311) -> (-184.116, -29.079)
  line L369 (-184.7432, -32.8122) -> (-185.3458, -32.4643)
  line L370 (-183.6779, -32.4915) -> (-181.5277, -28.7673)
  line L371 (-184.116, -29.079) -> (-186.2661, -32.8032)
  line L372 (-186.3866, -28.7039) -> (-185.784, -29.0518)
  line L373 (-180.9251, -29.1153) -> (-183.0752, -32.8394)
  line L374 (-185.3458, -32.4643) -> (-183.1957, -28.7401)
  line L375 (-183.1957, -28.7401) -> (-182.5931, -29.0881)
  line L376 (-186.3866, -28.7039) -> (-185.784, -29.0518)
  line L377 (-183.1957, -28.7401) -> (-182.5931, -29.0881)
  line L378 (-179.8118, -32.8172) -> (-180.4144, -32.4692)
  line L379 (-179.8118, -32.8172) -> (-180.4144, -32.4692)
  line L380 (-189.8199, -28.7076) -> (-189.2172, -29.0556)
  line L381 (-183.6779, -32.4915) -> (-181.5277, -28.7673)
  line L382 (-191.97, -32.4317) -> (-189.8199, -28.7076)
  line L383 (-178.2888, -32.8263) -> (-178.8915, -32.4783)
  line L384 (-190.7402, -29.0465) -> (-192.8903, -32.7706)
  line L385 (-184.116, -29.079) -> (-186.2661, -32.8032)
  line L386 (-191.3428, -28.6985) -> (-190.7402, -29.0465)
  line L387 (-183.0752, -32.8394) -> (-183.6779, -32.4915)
  line L388 (-181.5277, -28.7673) -> (-180.9251, -29.1153)
  line L389 (-189.6994, -32.8069) -> (-190.302, -32.4589)
  line L390 (-182.5931, -29.0881) -> (-184.7432, -32.8122)
  line L391 (-191.3674, -32.7797) -> (-191.97, -32.4317)
  line L392 (-191.3428, -28.6985) -> (-190.7402, -29.0465)
  line L393 (-194.5583, -32.7434) -> (-195.1609, -32.3955)
  line L394 (-179.3296, -29.0659) -> (-181.4798, -32.79)
  line L395 (-193.0108, -28.6714) -> (-192.4082, -29.0193)
  line L396 (-190.302, -32.4589) -> (-188.1519, -28.7348)
  line L397 (-179.3296, -29.0659) -> (-181.4798, -32.79)
  line L398 (-189.2172, -29.0556) -> (-191.3674, -32.7797)
  line L399 (-189.6994, -32.8069) -> (-190.302, -32.4589)
  line L400 (-187.9341, -32.776) -> (-188.5368, -32.428)
  line L401 (-192.8903, -32.7706) -> (-193.493, -32.4227)
  line L402 (-178.8915, -32.4783) -> (-176.7414, -28.7542)
  line L403 (-180.4144, -32.4692) -> (-178.2643, -28.7451)
  line L404 (-192.8903, -32.7706) -> (-193.493, -32.4227)
  line L405 (-170.5993, -32.538) -> (-168.4492, -28.8139)
  line L406 (-192.4082, -29.0193) -> (-194.5583, -32.7434)
  line L407 (-171.6401, -28.7777) -> (-171.0375, -29.1256)
  line L408 (-195.1609, -32.3955) -> (-193.0108, -28.6714)
  line L409 (-169.9967, -32.886) -> (-170.5993, -32.538)
  line L410 (-177.6617, -29.0931) -> (-179.8118, -32.8172)
  line L411 (-190.302, -32.4589) -> (-188.1519, -28.7348)
  line L412 (-192.4082, -29.0193) -> (-194.5583, -32.7434)
  line L413 (-179.9323, -28.7179) -> (-179.3296, -29.0659)
  line L414 (-193.0108, -28.6714) -> (-192.4082, -29.0193)
  line L415 (-167.8466, -29.1619) -> (-169.9967, -32.886)
  line L416 (-168.4492, -28.8139) -> (-167.8466, -29.1619)
  dimension "d30" = 6
  constraint perpendicular L6 L8
  constraint perpendicular L6 L9
  constraint perpendicular L6 L11
  constraint perpendicular L6 L13
  constraint parallel L13 L15
  constraint parallel L13 L17
  constraint perpendicular L17 L19
  constraint parallel L18 L20
  constraint perpendicular L17 L21
  constraint parallel L20 L22
  constraint perpendicular L17 L23
  constraint perpendicular L21 L25
  constraint parallel L25 L26
  constraint perpendicular L24 L27
  constraint parallel L8 L28
  constraint parallel L30 L31
  constraint parallel L28 L32
  constraint perpendicular L28 L33
  constraint parallel L33 L35
  constraint perpendicular L34 L36
  constraint parallel L1 L37
  constraint parallel L37 L38
  constraint parallel L38 L40
  constraint parallel L6 L42
  constraint parallel L6 L44
  constraint parallel L43 L45
  constraint parallel L44 L46
  constraint parallel L45 L47
  constraint parallel L46 L48
  constraint parallel L47 L49
  constraint perpendicular L46 L50
  constraint parallel L50 L52
  constraint perpendicular L47 L53
  constraint parallel L50 L54
  constraint parallel L0 L56
  constraint parallel L7 L58
  constraint parallel L58 L59
  constraint coincident A0.centre L61.end
  constraint horizontal L64
  constraint parallel L64 L65
  constraint parallel L61 L66
  constraint parallel L4 L67
  constraint perpendicular L8 L69
  constraint parallel L70 L72
  constraint parallel L72 L73
  constraint horizontal L74
  constraint parallel L9 L76
  constraint perpendicular L76 L77
  constraint parallel L77 L81
  constraint parallel L4 L83
  constraint parallel L4 L85
  constraint parallel L85 L87
  constraint parallel L64 L89
  constraint parallel L64 L90
  constraint parallel L64 L91
  constraint parallel L64 L93
  constraint parallel L94 L95
  constraint parallel L4 L96
  constraint perpendicular L94 L98
  constraint perpendicular L94 L99
  constraint parallel L54 L101
  constraint parallel L7 L103
  constraint perpendicular L48 L105
  constraint parallel L47 L107
  constraint parallel L48 L108
  constraint parallel L106 L109
  constraint parallel L48 L110
  constraint parallel L42 L112
  constraint perpendicular L106 L113
  constraint parallel L42 L114
  constraint parallel L106 L115
  constraint parallel L42 L116
  constraint perpendicular L115 L117
  constraint parallel L38 L118
  constraint parallel L116 L120
  constraint vertical L122
  constraint perpendicular L33 L125
  constraint parallel L124 L126
  constraint symmetric L124.start L127 L128.start
  constraint symmetric L124.end L127 L128.end
  constraint symmetric L125.end L127 L129.end
  constraint symmetric L126.end L127 L130.end
  constraint vertical L150
  constraint vertical L176
  constraint parallel L120 L178
  constraint parallel L178 L181
  constraint horizontal L183
  constraint vertical L184
  constraint horizontal L185
  constraint vertical L186
  constraint parallel L6 L188
  constraint horizontal L190
  constraint parallel L190 L192
  constraint parallel L192 L195
  constraint parallel L188 L197
  constraint parallel L188 L199
  constraint perpendicular L199 L200
  constraint perpendicular L200 L201
  constraint perpendicular L200 L203
  measures "d30" distance of L125.end L126.end
extrude "Extrude2" add sketch "Sketch2" along normal blind 2 contours L8 L28 L29 L30 L31 L32 L33 L34 L35 L36 L37 L38 L39 L40 L41 L42 L43 L44 L45 L46 L47 L48 L49 L50 L51 L52 L53 L54 L55 L56 L57 L58 L59 L60 L61 L62 L63 L64 L65 L66 L67 L68 L69 L70 L71 L72 L73 L74 L75 | L124 L125 L126 L128 L129 L130 | L131 L132 L133 L134 L135 L136 | L137 L138 L139 L141 L143 L146 | L140 L142 L144 L145 L147 L149 | L152 L154 L157 L160 L161 L168 | L153 L155 L158 L165 L170 L171 | L156 L159 L163 L164 L174 L175 | L166 L167 L169 L172 L173 L176 | L180 L181 L182 | L183 L184 L185 L186 | A12 | L187 L188 L189 L190 L191 L192 | L193 L194 L195 L196 | L197 L198 L199 L200 L201 L202 L203 L204 L205 L206 | L207 L208 L209 L210 L211 L212 L213 L214 | L215 L216 L217 L218 L219 L220 | L221 L229 L230 L232 L233 L234 | L222 L223 L224 L225 L226 L227 L228 L231 | L235 L239 L240 L241 L242 L248 | L236 L238 L247 L249 L259 L260 | L237 L243 L246 L250 L251 L257 | L244 L245 L252 L253 L254 L255 L256 L258 | L261 L266 L267 L272 L295 L306 | L262 L263 L278 L279 L282 L286 L290 L302 | L264 L265 L268 L281 L287 L296 | L269 L280 L283 L298 L311 L312 | L270 L271 L273 L274 L293 L294 L299 L309 | L275 L288 L291 L292 L307 L308 | L276 L297 L301 L303 L304 L305 | L277 L284 L285 L289 L300 L310 | L313 L314 L328 L345 L378 L379 L403 L410 | L315 L336 L338 L394 L397 L413 | L316 L341 L349 L354 L356 L357 L360 L407 | L317 L318 L342 L384 L386 L392 L401 L404 | L319 L320 L321 L335 L337 L346 | L322 L326 L331 L334 L348 L363 | L323 L333 L343 L358 L383 L402 | L324 L352 L361 L372 L376 L400 | L325 L330 L350 L351 L353 L355 | L327 L339 L359 L362 L366 L368 L371 L385 | L329 L340 L405 L409 L415 L416 | L332 L344 L389 L396 L399 L411 | L347 L365 L380 L382 L391 L398 | L364 L370 L373 L381 L387 L388 | L367 L369 L374 L375 L377 L390 | L393 L395 L406 L408 L412 L414 bodies 1
fillet "Fillet3" radius 1 3 edges at (-55, 48, 7) (-42, 29, 7) (-67, 29, 7) on bodies 1
fillet "Fillet4" radius 0.5 9 edges at (134.2833, 29.7167, 7) (135.1886, 29.1904, 7) (137.6491, 35, 7) (200, 36.377, 7) (200, 37.5655, 7) (182.5655, 36.377, 7) (178.2775, 35, 7) (182.1257, 37.5655, 7) (179, 34, 7) on bodies 1